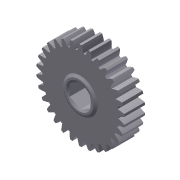
# Autodesk Inventor part: Spur Gear1
Saved by Autodesk Inventor 2015 (Build 190159000, 159)
## iProperties
Created: 2012-06-03
Part Number: Spur Gear1
Material: Aluminum-6061
Document SubType Name: Modeling
Designer: Nemo
Categories: <?xml version="1.0" encoding="UTF-16"?> <MemberInstance><Categories><FamilyTemplate><FamilyTemplateParameter ValueType="xs:double" Id="1" ObjectReferenceKey="da_z" ObjectType="kUserParameterObject"/><FamilyTemplateParameter ValueType="xs:double" Id="2" ObjectReferenceKey="da_b" ObjectType="kUserParameterObject"/><FamilyTemplateParameter ValueType="xs:double" Id="3" ObjectReferenceKey="da_beta" ObjectType="kUserParameterObject"/><FamilyTemplateParameter ValueType="xs:double" Id="4" ObjectReferenceKey="da_da" ObjectType="kUserParameterObject"/><FamilyTemplateParameter ValueType="xs:double" Id="5" ObjectReferenceKey="da_aw" ObjectType="kUserParameterObject"/><FamilyTemplateParameter ValueType="xs:string" Id="6" ObjectReferenceKey="EAIAABAAAAC/AAAAAAAAAIAAAAAAAAAA" ObjectType="83910656" SubObjectId="SurfaceGeometry"/></FamilyTemplate><ParamToTemplateMap><ParamToTemplate CategoryParameter="//CategoryParameter[@InternalName='046C89C9-8512-4d59-83FE-43B91F4F132A']" TemplateParameter="1"/><ParamToTemplate CategoryParameter="//CategoryParameter[@InternalName='2552DF32-E462-4b46-AEBF-C6C7768E72AC']" TemplateParameter="2"/><ParamToTemplate CategoryParameter="//CategoryParameter[@InternalName='C9EE641D-15FC-4fae-A226-E94C4372FDD7']" TemplateParameter="3"/><ParamToTemplate><ParamToTemplate CategoryParameter="//CategoryParameter[@InternalName='00B6519A-459B-49c7-AD84-2E56D39A5744']" ConstantValue="0.000000"/></ParamToTemplate><ParamToTemplate><ParamToTemplate CategoryParameter="//CategoryParameter[@InternalName='04B31F0E-C7A6-4894-AA32-9629BEFACF47']" ConstantValue="1.000000"/></ParamToTemplate><ParamToTemplate><ParamToTemplate CategoryParameter="//CategoryParameter[@InternalName='43CBEC2E-7847-49e7-A936-2F7889FCB2D9']" ConstantValue="0.250000"/></ParamToTemplate><ParamToTemplate><ParamToTemplate CategoryParameter="//CategoryParameter[@InternalName='B1EFC894-105D-4ebd-86BF-FA20ED196853']" ConstantValue="0.333500"/></ParamToTemplate><ParamToTemplate><ParamToTemplate CategoryParameter="//CategoryParameter[@InternalName='51175063-3D10-4879-93E8-6246FE8B403D']" ConstantValue="2060110000.000000"/></ParamToTemplate><ParamToTemplate><ParamToTemplate CategoryParameter="//CategoryParameter[@InternalName='A3A52E27-4454-46a9-B0BD-C932399B70AF']" ConstantValue="0.300000"/></ParamToTemplate><ParamToTemplate><ParamToTemplate CategoryParameter="//CategoryParameter[@InternalName='91B76062-C214-41d9-B1B9-14D2AB99603D']" ConstantValue="0.127000"/></ParamToTemplate><ParamToTemplate><ParamToTemplate CategoryParameter="//CategoryParameter[@InternalName='374E806E-8B8A-4dda-A9AA-1039D6500AD2']" ConstantValue="7.874016"/></ParamToTemplate><ParamToTemplate><ParamToTemplate CategoryParameter="//CategoryParameter[@InternalName='2D373A89-B862-43d6-8D0B-0CBF12AB9F6C']" ConstantValue="0.253073"/></ParamToTemplate><ParamToTemplate CategoryParameter="//CategoryParameter[@InternalName='37777632-D6A2-4fac-9D53-DB8ACD95C989']" TemplateParameter="4"/><ParamToTemplate CategoryParameter="//CategoryParameter[@InternalName='FD1017F1-B727-4f7e-9707-0F86F1FF9423']" TemplateParameter="5"/><ParamToTemplate><ParamToTemplate CategoryParameter="//CategoryParameter[@InternalName='9E1B4470-B2D3-4ff1-B813-535BB4CDF51A']" ConstantValue="3520790.000000"/></ParamToTemplate><ParamToTemplate><ParamToTemplate CategoryParameter="//CategoryParameter[@InternalName='F8452263-BFF6-458c-9FB1-07C4B99E95CD']" ConstantValue="11389170.000000"/></ParamToTemplate><ParamToTemplate><ParamToTemplate CategoryParameter="//CategoryParameter[@InternalName='3E3BB259-FD49-497f-8171-6EBC954A3479']" ConstantValue="2.000000"/></ParamToTemplate><ParamToTemplate CategoryParameter="//CategoryParameter[@InternalName='27C3BAF2-7550-4e4b-AE2C-0DB134B7D9B7']" TemplateParameter="6"/></ParamToTemplateMap><Category DisplayName="Gear" InternalName="DC85795E-93AB-48d5-8EEE-5A27447B64BD" Mnemonic="Gear"><CategoryParameter DisplayName="z" InternalName="046C89C9-8512-4d59-83FE-43B91F4F132A" Mnemonic="z"/><CategoryParameter DisplayName="b" InternalName="2552DF32-E462-4b46-AEBF-C6C7768E72AC" Mnemonic="b"/><CategoryParameter DisplayName="||b|" InternalName="C9EE641D-15FC-4fae-A226-E94C4372FDD7" Mnemonic="beta"/><CategoryParameter DisplayName="x" InternalName="00B6519A-459B-49c7-AD84-2E56D39A5744" Mnemonic="x"/><CategoryParameter DisplayName="a*" InternalName="04B31F0E-C7A6-4894-AA32-9629BEFACF47" Mnemonic="a"/><CategoryParameter DisplayName="c*" InternalName="43CBEC2E-7847-49e7-A936-2F7889FCB2D9" Mnemonic="c"/><CategoryParameter DisplayName="r|.f|*" InternalName="B1EFC894-105D-4ebd-86BF-FA20ED196853" Mnemonic="rf"/><CategoryParameter DisplayName="E" InternalName="51175063-3D10-4879-93E8-6246FE8B403D" Mnemonic="E"/><CategoryParameter DisplayName="||m|" InternalName="A3A52E27-4454-46a9-B0BD-C932399B70AF" Mnemonic="mi"/><Category DisplayName="SpurGear" InternalName="26C5A22E-A91E-4dfd-A3B3-23CCAFAE1764" Mnemonic="SpurGear"><CategoryParameter DisplayName="m" InternalName="91B76062-C214-41d9-B1B9-14D2AB99603D" Mnemonic="m"/><CategoryParameter DisplayName="P" InternalName="374E806E-8B8A-4dda-A9AA-1039D6500AD2" Mnemonic="PP"/><CategoryParameter DisplayName="||a|" InternalName="2D373A89-B862-43d6-8D0B-0CBF12AB9F6C" Mnemonic="alpha"/><CategoryParameter DisplayName="d|.a|" InternalName="37777632-D6A2-4fac-9D53-DB8ACD95C989" Mnemonic="da"/><CategoryParameter DisplayName="a|.w|" InternalName="FD1017F1-B727-4f7e-9707-0F86F1FF9423" Mnemonic="aw"/><CategoryParameter DisplayName="||s||.Flim|" InternalName="9E1B4470-B2D3-4ff1-B813-535BB4CDF51A" Mnemonic="sFlim"/><CategoryParameter DisplayName="||s||.Hlim|" InternalName="F8452263-BFF6-458c-9FB1-07C4B99E95CD" Mnemonic="sHlim"/><CategoryParameter DisplayName="type" InternalName="3E3BB259-FD49-497f-8171-6EBC954A3479" Mnemonic="type"/><CategoryParameter DisplayName="PitchDiameter" InternalName="27C3BAF2-7550-4e4b-AE2C-0DB134B7D9B7" Mnemonic="IDS_PITCHDIAM"/></Category></Category></Categories></MemberInstance>
Density: 2.71 g/cm^3
Mass: 29.2157 g
Surface Area: 45.6064 cm^2
Volume: 10.7807 cm^3
Appearance: Aluminum - Flat
CustomPartVersion: 1
Author: Nemo
Autodesk Inventor part; units mm, degrees
sketch "Sketch1" plane through (0, 0, 0) normal (0, 0, 1) x (1, 0, 0)
  circle A0 centre (0, 0) radius 20.32
  dimension "d0" = 40.64
  constraints: 1 centre point
  measures "d0" diameter of A0
extrude "Extrusion1" add sketch "Sketch1" along normal blind 9.525
sketch "Sketch2" plane through (0, 0, 0) normal (0, 0, -1) x (-1, 0, 0)
  circle A0 centre (0, 0) radius 20.32 projected
  circle A1 centre (0, 0) radius 19.05
  dimension "d3" = 38.1
  constraints: 1 centre point, 1 coincident
  measures "d3" diameter of A1
surface extrude "Pitch Diameter" sketch "Sketch2" against normal through all shown no curves A1
ref_plane "Work Plane1" through (0, 0, 0) normal (1, 0, 0) x (0, 1, 0)
ref_plane "Work Plane2" through (0, 0, 0) normal (0.9945219, 0.1045285, 0) x (0, 0, 1)
ref_plane "Work Plane3" through (0, 0, 4.7625) normal (0, 0, -1) x (-1, 0, 0)
spur gear teeth "Spur Gear" teeth 30 pitch diameter 38.1 tip diameter 40.64 root diameter 34.925 face width 9.525 start plane through (0, 0, 0) normal (0, 0, -1) x (-1, 0, 0)
sketch "Sketch3" plane through (0, 0, 9.525) normal (0, 0, 1) x (1, 0, 0)
  arc A0 (-3.703, 19.9797) -> (-4.7436, 19.7586) centre (0, 0) ccw projected
  circle A1 centre (0, 0) radius 7.9502
  dimension "d20" = 15.9004
  constraints: 1 centre point, 1 coincident
  measures "d20" diameter of A1
extrude "Extrusion2" add sketch "Sketch3" along normal blind 0.635
sketch "Sketch4" plane through (0, 0, 10.16) normal (0, 0, 1) x (1, 0, 0)
  circle A0 centre (0, 0) radius 7.9502 projected
  line L0 (0, 5.4993) -> (4.7625, 2.7496)
  line L1 (4.7625, 2.7496) -> (4.7625, -2.7496)
  line L2 (4.7625, -2.7496) -> (0, -5.4993)
  line L3 (0, -5.4993) -> (-4.7625, -2.7496)
  line L4 (-4.7625, -2.7496) -> (-4.7625, 2.7496)
  line L5 (-4.7625, 2.7496) -> (0, 5.4993)
  dimension "d23" = 9.525
  constraints: 12 end point, 1 coincident, 1 vertical alignment, 13 other
  measures "d23" distance between parallel lines of L1 L4
extrude "Extrusion3" cut sketch "Sketch4" against normal through all contours L0 L1 L2 L3 L4 L5
sketch "Sketch5" plane through (0, 0, 0) normal (1, 0, 0) x (0, 1, 0)
  line L0 (-7.9502, 9.525) -> (-7.9502, 10.16) projected
  line L1 (-7.9502, 10.16) -> (-5.4993, 10.16) projected
  line L2 (-5.4993, 10.16) -> (-5.4993, 0) projected
  line L3 (-5.4993, 0) -> (-20.32, 0) projected
  line L4 (-20.32, 0) -> (-20.32, 9.525) projected
  line L5 (-20.32, 9.525) -> (-7.9502, 9.525) projected
  line L6 (7.9502, 10.16) -> (7.9502, 9.525) projected
  line L7 (7.9502, 9.525) -> (20.32, 9.525) projected
  line L8 (20.32, 9.525) -> (20.32, 0) projected
  line L9 (20.32, 0) -> (5.4993, 0) projected
  line L10 (5.4993, 0) -> (5.4993, 10.16) projected
  line L11 (5.4993, 10.16) -> (7.9502, 10.16) projected
  line L12 (0, 0) -> (0, 16.7192)
  line L13 (7.9502, 9.525) -> (6.8072, 10.16)
  line L14 (6.8072, 10.16) -> (7.9502, 10.16)
  line L15 (7.9502, 10.16) -> (7.9502, 9.525)
  line L16 (5.9182, 10.16) -> (3.6977, 8.9266)
  line L17 (3.6977, 8.9266) -> (3.6977, 10.16)
  line L18 (3.6977, 10.16) -> (5.9182, 10.16)
  dimension "d26" = 1.143
  dimension "d27" = 0.889
  dimension "d28" = 29.05
  dimension "d29" = 2.54
  constraints: 14 end point, 2 collinear, 2 perpendicular, 2 point on line, 1 parallel
  measures "d26" distance of L13.end L6.start
  measures "d27" distance of L16.start L13.end
  measures "d28" angle of L16 L18
  measures "d29" distance of L16.start L16.end
revolve "Revolution1" cut sketch "Sketch5" angle 360 about axis through (0, 0, 0) along (0, 0, 1) contours L6 L13 L11 | L16 L10 L11 | L10 L16 L17 L18
equation "\"d0\" = da_da"
equation "\"d1\" = da_b"
equation "\"d3\" = da_dw"
equation "\"d15\" = da_aw"
equation "\"d19\" = da_aw"
equation "\"da_da\" = 40.64"
equation "\"da_b\" = 9.525"
equation "\"da_dw\" = 38.1"
equation "\"da_aw\" = 95.25"
body "Solid1"
body "Srf1"
